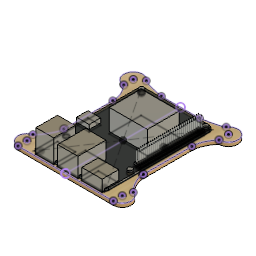
Maaxboard mounted (Autodesk Fusion 360 design; units mm, degrees)
part number: 2026-02-05-11-10-26-845
Autodesk Fusion 360 part; units mm, degrees
sketch "Mount board" plane through (0, 0, 0) normal (0, 0, 1) x (1, 0, 0)
  line L0 (-37.35, 0) -> (37.35, 0)
  line L1 (-31, 90) -> (31, 90)
  line L2 (0, 90) -> (0, 0)
  line L3 (-31, 90) -> (-31, 0)
  line L4 (31, 90) -> (31, 0)
  arc A0 (-39.3579, 13.7058) -> (-37.35, 0) centre (-37.35, 7) ccw
  spline S0 degree 5 poles (-39.3579, 13.7058) (-39.0766, 13.9227) (-38.5354, 14.3685) (-37.7884, 15.0728) (-36.908, 16.081) (-35.9311, 17.4458) (-35.003, 18.9053) (-34.0689, 20.4546) (-33.1263, 22.0975) (-32.2391, 23.848) (-31.5041, 25.7261) (-31.1237, 27.3492) (-30.9957, 28.6435) (-30.986, 29.5419) (-31, 30) knots 0 0 0 0 0 0 0.1 0.2 0.3 0.4 0.5 0.6 0.7 0.8 0.9 1 1 1 1 1 1
  circle A1 centre (-37.35, 7) radius 1.4
  arc A2 (37.35, 0) -> (39.3579, 13.7058) centre (37.35, 7) ccw
  spline S1 degree 5 poles (39.3579, 13.7058) (39.0766, 13.9227) (38.5354, 14.3685) (37.7884, 15.0728) (36.908, 16.081) (35.9311, 17.4458) (35.003, 18.9053) (34.0689, 20.4546) (33.1263, 22.0975) (32.2391, 23.848) (31.5041, 25.7261) (31.1237, 27.3492) (30.9957, 28.6435) (30.986, 29.5419) (31, 30) knots 0 0 0 0 0 0 0.1 0.2 0.3 0.4 0.5 0.6 0.7 0.8 0.9 1 1 1 1 1 1
  line L5 (-40.9476, 12.4803) -> (-37.7683, 14.9314)
  line L6 (-30.9328, 27.8077) -> (-31.0672, 32.1923)
  line L7 (40.9476, 12.4803) -> (37.7683, 14.9314)
  line L8 (30.9328, 27.8077) -> (31.0672, 32.1923)
  circle A3 centre (37.35, 7) radius 1.4
  circle A4 centre (-37.35, 90.3) radius 1.4
  circle A5 centre (-37.35, 90.3) radius 7.4
  spline S2 degree 5 poles (-37.35, 82.9) (-37.1115, 82.6183) (-36.6442, 82.0534) (-35.972, 81.2012) (-35.1342, 80.0554) (-34.1911, 78.606) (-33.3621, 77.1379) (-32.6571, 75.6494) (-32.083, 74.1394) (-31.6366, 72.6084) (-31.3088, 71.0579) (-31.1342, 69.8032) (-31.0494, 68.8545) (-31.0131, 68.2187) (-31, 67.9) knots 0 0 0 0 0 0 0.1 0.2 0.3 0.4 0.5 0.6 0.7 0.8 0.9 1 1 1 1 1 1
  line L9 (-37.35, 82.9) -> (-31, 82.9) construction
  line L10 (-31, 82.9) -> (-31, 67.9) construction
  line L11 (-34.175, 82.9) -> (-31, 82.9) construction
  spline S3 degree 5 poles (-31.2889, 94.5453) (-31.193, 94.4644) (-30.9783, 94.3016) (-30.5874, 94.0544) (-29.9264, 93.7188) (-28.8549, 93.2886) (-27.5267, 92.8473) (-25.9435, 92.3949) (-24.1262, 91.9324) (-22.1003, 91.4609) (-19.891, 90.9814) (-17.9926, 90.5921) (-16.5005, 90.2972) (-15.4759, 90.0993) (-14.9561, 90) knots 0 0 0 0 0 0 0.1 0.2 0.3 0.4 0.5 0.6 0.7 0.8 0.9 1 1 1 1 1 1
  spline S4 degree 5 poles (37.35, 82.9) (37.1115, 82.6183) (36.6442, 82.0534) (35.972, 81.2012) (35.1342, 80.0554) (34.1911, 78.606) (33.3621, 77.1379) (32.6571, 75.6494) (32.083, 74.1394) (31.6366, 72.6084) (31.3088, 71.0579) (31.1342, 69.8032) (31.0494, 68.8545) (31.0131, 68.2187) (31, 67.9) knots 0 0 0 0 0 0 0.1 0.2 0.3 0.4 0.5 0.6 0.7 0.8 0.9 1 1 1 1 1 1
  line L12 (-38.5735, 84.3453) -> (-36.1265, 81.4547)
  line L13 (-31.0729, 69.6717) -> (-30.9271, 66.1283)
  line L14 (38.5735, 84.3453) -> (36.1265, 81.4547)
  line L15 (31.0729, 69.6717) -> (30.9271, 66.1283)
  circle A6 centre (37.35, 90.3) radius 7.4
  circle A7 centre (37.35, 90.3) radius 1.4
  spline S5 degree 5 poles (31.2889, 94.5453) (31.193, 94.4644) (30.9783, 94.3016) (30.5874, 94.0544) (29.9264, 93.7188) (28.8549, 93.2886) (27.5267, 92.8473) (25.9435, 92.3949) (24.1262, 91.9324) (22.1003, 91.4609) (19.891, 90.9814) (17.9926, 90.5921) (16.5005, 90.2972) (15.4759, 90.0993) (14.9561, 90) knots 0 0 0 0 0 0 0.1 0.2 0.3 0.4 0.5 0.6 0.7 0.8 0.9 1 1 1 1 1 1
  line L16 (-32.1151, 95.2425) -> (-30.4626, 93.8481)
  line L17 (-17.1383, 90.4168) -> (-12.7739, 89.5832)
  line L18 (32.1151, 95.2425) -> (30.4626, 93.8481)
  line L19 (17.1383, 90.4168) -> (12.7739, 89.5832)
  point P0 (0, 90)
  point P1 (-34.35, 20)
  point P2 (34.35, 20)
  point P3 (-32.5875, 75.4)
  point P4 (-34.175, 82.9)
  point P5 (-31, 75.4)
  point P6 (-32.5875, 82.9)
  point P7 (-27.9561, 93)
  point P8 (-29.9561, 90)
  point P9 (32.5875, 75.4)
  point P10 (27.9561, 93)
  dimension "d1" = 74.7
  dimension "d2" = 62
  dimension "d3" = 90
  dimension "d4" = 7
  dimension "d5" = 30
  dimension "d6" = 20
  dimension "d7" = 3
  dimension "d8" = 2.8
  dimension "d9" = 2.8
  dimension "d10" = 83.3
  dimension "d11" = 14.8
  dimension "d12" = 15
  dimension "d13" = 15
  dimension "d14" = 3
  dimension "d15" = 2
  constraint horizontal L0
  constraint midpoint L0 L2.end
  constraint coincident L2.end origin
  constraint horizontal L1
  constraint midpoint L1 P0
  constraint coincident P0 L2.start
  constraint coincident L0 L3.end
  constraint perpendicular L0 L3
  constraint coincident L0 L4.end
  constraint perpendicular L0 L4
  constraint tangent L0 A0
  constraint coincident L3 S0.end
  constraint perpendicular L0 L2
  constraint concentric A0 A1
  constraint midpoint A0.start L5
  constraint midpoint S0.end L6
  constraint symmetric L0.start L2 L0.end
  constraint symmetric L2 A0.start A2.end
  constraint symmetric L2 A0 A2
  constraint symmetric L2 P1 P2
  constraint symmetric L2 S0.end S1.end
  constraint symmetric L2 A1 A3
  constraint symmetric L2 L5.start L7.start
  constraint symmetric L2 L5.end L7.end
  constraint symmetric L2 L6.start L8.start
  constraint symmetric L2 L6.end L8.end
  constraint concentric A4 A5
  constraint vertical A0.centre A4.centre
  constraint coincident A5 S2.start
  constraint coincident L3 S2.end
  constraint vertical A4.centre S2.start
  constraint coincident L3 L9.end
  constraint tangent A5 L9
  constraint midpoint L10 P5
  constraint horizontal P3 P5
  constraint coincident P4 L11.start
  constraint perpendicular L3 L11
  constraint midpoint L11 P6
  constraint vertical P3 P6
  constraint coincident A5 S3.start
  constraint coincident L1 S3.end
  constraint coincident L1 P8
  constraint coincident A5 P8
  constraint midpoint S2.start L12
  constraint midpoint S2.end L13
  constraint midpoint S3.start L16
  constraint midpoint S3.end L17
  constraint symmetric L2 A4 A7
  constraint symmetric L2 A5 A6
  constraint symmetric L2 S2.start S4.start
  constraint symmetric L2 P3 P9
  constraint symmetric L2 S2.end S4.end
  constraint symmetric L2 S3.start S5.start
  constraint symmetric L2 P7 P10
  constraint symmetric L2 S3.end S5.end
  constraint symmetric L2 L12.start L14.start
  constraint symmetric L2 L12.end L14.end
  constraint symmetric L2 L13.start L15.start
  constraint symmetric L2 L13.end L15.end
  constraint symmetric L2 L16.start L18.start
  constraint symmetric L2 L16.end L18.end
  constraint symmetric L2 L17.start L19.start
  constraint symmetric L2 L17.end L19.end
  measures "d1" distance of L0.start L0.end
  measures "d2" distance of L1.start L1.end
  measures "d3" distance of L0.start L1
  measures "d4" radius of A0
  measures "d5" distance of L3.end S0.end
  measures "d6" vertical distance of L3.end P1
  measures "d7" horizontal distance of L0.start P1
  measures "d8" diameter of A1
  measures "d9" diameter of A4
  measures "d10" vertical distance of A0.centre A4.centre
  measures "d11" diameter of A5
  measures "d12" distance of S2.end L9.end
  measures "d13" distance of S3.end P8
  measures "d14" vertical distance of P7 P8
  measures "d15" horizontal distance of P7 P8
extrude "Extrude1" add sketch "Mount board" along normal blind 3 contours L0 L3 A0 S0 | L0 L1 L2 L3 S0 A5 | L0 L1 L2 L4 S1 A6 | L0 L4 A2 S1 | L1 A5 S3 | L1 A6 S5 | L3 A5 S2 | L1 L3 A5 | L1 L3 A5 | L1 L4 A6 | L1 L4 A6 | L4 S4 A6 makes body 1
sketch "Sketch2" plane through (0, 0, 3) normal (0, 0, 1) x (-1, 0, 0)
  circle A0 centre (37.35, -90.3) radius 1.4
  circle A1 centre (-37.35, -90.3) radius 1.4
  circle A2 centre (37.35, -7) radius 1.4
  circle A3 centre (-37.35, -7) radius 1.4
  arc A4 (-37.35, -82.9) -> (-31.2889, -94.5453) centre (-37.35, -90.3) ccw
  spline S0 degree 5 poles (-31.2889, -94.5453) (-31.193, -94.4644) (-30.9783, -94.3016) (-30.5874, -94.0544) (-29.9264, -93.7188) (-28.8549, -93.2886) (-27.5267, -92.8473) (-25.9435, -92.3949) (-24.1262, -91.9324) (-22.1003, -91.4609) (-19.891, -90.9814) (-17.9926, -90.5921) (-16.5005, -90.2972) (-15.4759, -90.0993) (-14.9561, -90) knots 0 0 0 0 0 0 0.1 0.2 0.3 0.4 0.5 0.6 0.7 0.8 0.9 1 1 1 1 1 1
  line L0 (-14.9561, -90) -> (14.9561, -90)
  spline S1 degree 5 poles (14.9561, -90) (15.4759, -90.0993) (16.5005, -90.2972) (17.9926, -90.5921) (19.891, -90.9814) (22.1003, -91.4609) (24.1262, -91.9324) (25.9435, -92.3949) (27.5267, -92.8473) (28.8549, -93.2886) (29.9264, -93.7188) (30.5874, -94.0544) (30.9783, -94.3016) (31.193, -94.4644) (31.2889, -94.5453) knots -1 -1 -1 -1 -1 -1 -0.9 -0.8 -0.7 -0.6 -0.5 -0.4 -0.3 -0.2 -0.1 0 0 0 0 0 0
  arc A5 (31.2889, -94.5453) -> (37.35, -82.9) centre (37.35, -90.3) ccw
  spline S2 degree 5 poles (37.35, -82.9) (37.1115, -82.6183) (36.6442, -82.0534) (35.972, -81.2012) (35.1342, -80.0554) (34.1911, -78.606) (33.3621, -77.1379) (32.6571, -75.6494) (32.083, -74.1394) (31.6366, -72.6084) (31.3088, -71.0579) (31.1342, -69.8032) (31.0494, -68.8545) (31.0131, -68.2187) (31, -67.9) knots 0 0 0 0 0 0 0.1 0.2 0.3 0.4 0.5 0.6 0.7 0.8 0.9 1 1 1 1 1 1
  line L1 (31, -67.9) -> (31, -30)
  spline S3 degree 5 poles (31, -30) (30.9948, -29.8295) (30.9922, -29.6602) (30.9922, -29.4921) (30.9948, -29.3252) (31, -29.1596) knots -1 -1 -1 -1 -1 -1 -0.962773 -0.962773 -0.962773 -0.962773 -0.962773 -0.962773
  spline S4 degree 5 poles (31, -29.1596) (31.0088, -28.8804) (31.0505, -28.1652) (31.1963, -27.0481) (31.5588, -25.5863) (32.2391, -23.848) (33.1263, -22.0975) (34.0689, -20.4546) (35.003, -18.9053) (35.9311, -17.4458) (36.908, -16.081) (37.7884, -15.0728) (38.5354, -14.3685) (39.0766, -13.9227) (39.3579, -13.7058) knots -0.962773 -0.962773 -0.962773 -0.962773 -0.962773 -0.962773 -0.9 -0.8 -0.7 -0.6 -0.5 -0.4 -0.3 -0.2 -0.1 0 0 0 0 0 0
  arc A6 (39.3579, -13.7058) -> (37.35, 0) centre (37.35, -7) ccw
  line L2 (37.35, 0) -> (-37.35, 0)
  arc A7 (-37.35, 0) -> (-39.3579, -13.7058) centre (-37.35, -7) ccw
  spline S5 degree 5 poles (-39.3579, -13.7058) (-39.0766, -13.9227) (-38.5354, -14.3685) (-37.7884, -15.0728) (-36.908, -16.081) (-35.9311, -17.4458) (-35.003, -18.9053) (-34.0689, -20.4546) (-33.1263, -22.0975) (-32.2391, -23.848) (-31.5588, -25.5863) (-31.1963, -27.0481) (-31.0505, -28.1652) (-31.0088, -28.8804) (-31, -29.1596) knots 0 0 0 0 0 0 0.1 0.2 0.3 0.4 0.5 0.6 0.7 0.8 0.9 0.962773 0.962773 0.962773 0.962773 0.962773 0.962773
  spline S6 degree 5 poles (-31, -29.1596) (-30.9948, -29.3252) (-30.9922, -29.4921) (-30.9922, -29.6602) (-30.9948, -29.8295) (-31, -30) knots 0.962773 0.962773 0.962773 0.962773 0.962773 0.962773 1 1 1 1 1 1
  line L3 (-31, -30) -> (-31, -67.9)
  spline S7 degree 5 poles (-31, -67.9) (-31.0131, -68.2187) (-31.0494, -68.8545) (-31.1342, -69.8032) (-31.3088, -71.0579) (-31.6366, -72.6084) (-32.083, -74.1394) (-32.6571, -75.6494) (-33.3621, -77.1379) (-34.1911, -78.606) (-35.1342, -80.0554) (-35.972, -81.2012) (-36.6442, -82.0534) (-37.1115, -82.6183) (-37.35, -82.9) knots -1 -1 -1 -1 -1 -1 -0.9 -0.8 -0.7 -0.6 -0.5 -0.4 -0.3 -0.2 -0.1 0 0 0 0 0 0
  line L4 (0, -90) -> (0, 0)
  line L5 (-25.1, -87.5) -> (25.1, -87.5)
  line L6 (28.1, -84.5) -> (28.1, -5.5)
  line L7 (25.1, -2.5) -> (-25.1, -2.5)
  line L8 (-28.1, -5.5) -> (-28.1, -84.5)
  line L9 (-28.1, -87.5) -> (28.1, -2.5) construction
  line L10 (28.1, -87.5) -> (-28.1, -2.5) construction
  arc A8 (25.1, -87.5) -> (28.1, -84.5) centre (25.1, -84.5) ccw
  arc A9 (-28.1, -84.5) -> (-25.1, -87.5) centre (-25.1, -84.5) ccw
  arc A10 (-25.1, -2.5) -> (-28.1, -5.5) centre (-25.1, -5.5) ccw
  arc A11 (28.1, -5.5) -> (25.1, -2.5) centre (25.1, -5.5) ccw
  circle A12 centre (25.1, -84.5) radius 1.875
  circle A13 centre (-25.1, -84.5) radius 1.875
  line L11 (-22.1, -81.5) -> (-22.1, -31.5)
  line L12 (-22.1, -31.5) -> (-27.1, -31.5)
  line L13 (-27.1, -31.5) -> (-27.1, -81.5)
  circle A14 centre (-25.85, -80.7753) radius 0.335
  line L14 (-22.1, -81.5) -> (-24.6, -81.5)
  line L15 (-24.6, -81.5) -> (-27.1, -81.5)
  circle A15 centre (-23.35, -80.7753) radius 0.335
  circle A16 centre (-25.85, -79.2108) radius 0.335
  circle A17 centre (-23.35, -79.2108) radius 0.335
  circle A18 centre (-25.85, -77.6463) radius 0.335
  circle A19 centre (-23.35, -77.6463) radius 0.335
  circle A20 centre (-25.85, -76.0818) radius 0.335
  circle A21 centre (-23.35, -76.0818) radius 0.335
  circle A22 centre (-25.85, -74.5173) radius 0.335
  circle A23 centre (-23.35, -74.5173) radius 0.335
  circle A24 centre (-25.85, -72.9528) radius 0.335
  circle A25 centre (-23.35, -72.9528) radius 0.335
  circle A26 centre (-25.85, -71.3882) radius 0.335
  circle A27 centre (-23.35, -71.3882) radius 0.335
  circle A28 centre (-25.85, -69.8237) radius 0.335
  circle A29 centre (-23.35, -69.8237) radius 0.335
  circle A30 centre (-25.85, -68.2592) radius 0.335
  circle A31 centre (-23.35, -68.2592) radius 0.335
  circle A32 centre (-25.85, -66.6947) radius 0.335
  circle A33 centre (-23.35, -66.6947) radius 0.335
  circle A34 centre (-25.85, -65.1302) radius 0.335
  circle A35 centre (-23.35, -65.1302) radius 0.335
  circle A36 centre (-25.85, -63.5657) radius 0.335
  circle A37 centre (-23.35, -63.5657) radius 0.335
  circle A38 centre (-25.85, -62.0012) radius 0.335
  circle A39 centre (-23.35, -62.0012) radius 0.335
  circle A40 centre (-25.85, -60.4366) radius 0.335
  circle A41 centre (-23.35, -60.4366) radius 0.335
  circle A42 centre (-25.85, -58.8721) radius 0.335
  circle A43 centre (-23.35, -58.8721) radius 0.335
  circle A44 centre (-25.85, -57.3076) radius 0.335
  circle A45 centre (-23.35, -57.3076) radius 0.335
  circle A46 centre (-25.85, -55.7431) radius 0.335
  circle A47 centre (-23.35, -55.7431) radius 0.335
  circle A48 centre (-25.85, -54.1786) radius 0.335
  circle A49 centre (-23.35, -54.1786) radius 0.335
  circle A50 centre (-25.85, -52.6141) radius 0.335
  circle A51 centre (-23.35, -52.6141) radius 0.335
  circle A52 centre (-25.85, -51.0495) radius 0.335
  circle A53 centre (-23.35, -51.0495) radius 0.335
  circle A54 centre (-25.85, -49.485) radius 0.335
  circle A55 centre (-23.35, -49.485) radius 0.335
  circle A56 centre (-25.85, -47.9205) radius 0.335
  circle A57 centre (-23.35, -47.9205) radius 0.335
  circle A58 centre (-25.85, -46.356) radius 0.335
  circle A59 centre (-23.35, -46.356) radius 0.335
  circle A60 centre (-25.85, -44.7915) radius 0.335
  circle A61 centre (-23.35, -44.7915) radius 0.335
  circle A62 centre (-25.85, -43.227) radius 0.335
  circle A63 centre (-23.35, -43.227) radius 0.335
  circle A64 centre (-25.85, -41.6624) radius 0.335
  circle A65 centre (-23.35, -41.6624) radius 0.335
  circle A66 centre (-25.85, -40.0979) radius 0.335
  circle A67 centre (-23.35, -40.0979) radius 0.335
  circle A68 centre (-25.85, -38.5334) radius 0.335
  circle A69 centre (-23.35, -38.5334) radius 0.335
  circle A70 centre (-25.85, -36.9689) radius 0.335
  circle A71 centre (-23.35, -36.9689) radius 0.335
  circle A72 centre (-25.85, -35.4044) radius 0.335
  circle A73 centre (-23.35, -35.4044) radius 0.335
  circle A74 centre (-25.85, -33.8399) radius 0.335
  circle A75 centre (-23.35, -33.8399) radius 0.335
  circle A76 centre (-25.85, -32.2753) radius 0.335
  circle A77 centre (-23.35, -32.2753) radius 0.335
  line L16 (-20.1, -69) -> (9.9, -69)
  line L17 (9.9, -69) -> (9.9, -44)
  line L18 (9.9, -44) -> (-20.1, -44)
  line L19 (-20.1, -44) -> (-20.1, -69)
  line L20 (29.1, -46.5) -> (19.1, -46.5)
  line L21 (19.1, -46.5) -> (19.1, -37.5)
  line L22 (19.1, -37.5) -> (29.1, -37.5)
  line L23 (29.1, -37.5) -> (29.1, -46.5)
  line L24 (-27.1, -14.5) -> (-11.1, -14.5)
  line L25 (-11.1, -14.5) -> (-11.1, -1.5)
  line L26 (-11.1, -1.5) -> (-27.1, -1.5)
  line L27 (-27.1, -1.5) -> (-27.1, -14.5)
  line L28 (-8.1, -1.5) -> (7.9, -1.5)
  line L29 (7.9, -1.5) -> (7.9, -23.5)
  line L30 (7.9, -23.5) -> (-8.1, -23.5)
  line L31 (-8.1, -23.5) -> (-8.1, -1.5)
  line L32 (10.9, -1.5) -> (24.9, -1.5)
  line L33 (24.9, -1.5) -> (24.9, -18.5)
  line L34 (24.9, -18.5) -> (10.9, -18.5)
  line L35 (10.9, -18.5) -> (10.9, -1.5)
  circle A78 centre (-25.1, -25.5) radius 1.875
  circle A79 centre (25.1, -25.5) radius 1.875
  point P0 (0, -45)
  point P1 (0, -45)
  point P2 (-24.6, -81.5)
  point P3 (-23.35, -81.5)
  point P4 (-25.85, -81.5)
  point P5 (-20.1, -56.5)
  point P6 (-22.1, -56.5)
  dimension "d18" = 56.2
  dimension "d19" = 85
  dimension "d20" = 3
  dimension "d22" = 5
  dimension "d23" = 50
  dimension "d25" = 1
  dimension "d26" = 0.67
  dimension "d27" = 0.67
  dimension "d28" = 0.7247
  dimension "d29" = 3
  dimension "d32" = 0
  dimension "d33" = 48.5
  dimension "d34" = 30
  dimension "d35" = 25
  dimension "d36" = 2
  dimension "d37" = 10
  dimension "d38" = 9
  dimension "d39" = 1
  dimension "d40" = 35
  dimension "d41" = 1
  dimension "d42" = 16
  dimension "d43" = 1
  dimension "d44" = 13
  dimension "d45" = 16
  dimension "d46" = 22
  dimension "d48" = 14
  dimension "d49" = 17
  dimension "d50" = 3
  dimension "d51" = 3
  dimension "d52" = 23
  dimension "d53" = 3.75
  constraint midpoint L4 P1
  constraint horizontal L5
  constraint perpendicular L5 L6
  constraint parallel L5 L7
  constraint parallel L6 L8
  constraint coincident L9 P1
  constraint coincident L10 P1
  constraint coincident P1 P0
  constraint coincident L10.start L5
  constraint coincident L10.start L6
  constraint tangent L5 A8
  constraint tangent L6 A8
  constraint coincident L9.start L5
  constraint coincident L9.start L8
  constraint tangent L5 A9
  constraint tangent L8 A9
  constraint equal A8 A9
  constraint coincident L10.end L8
  constraint coincident L10.end L7
  constraint tangent L8 A10
  constraint tangent L7 A10
  constraint equal A8 A10
  constraint coincident L9.end L6
  constraint coincident L9.end L7
  constraint tangent L6 A11
  constraint tangent L7 A11
  constraint equal A8 A11
  constraint concentric A8 A12
  constraint concentric A9 A13
  constraint vertical L11
  constraint horizontal L12
  constraint vertical L13
  constraint coincident P2 L14.end
  constraint midpoint L14 P3
  constraint midpoint L15 P4
  constraint vertical A14.centre P4
  constraint vertical P3 A15.centre
  constraint horizontal A14.centre A15.centre
  constraint perpendicular L11 L14
  constraint perpendicular L13 L15
  constraint equal L14 L15
  constraint horizontal L16
  constraint vertical L17
  constraint horizontal L18
  constraint vertical L19
  constraint midpoint L19 P5
  constraint midpoint L11 P6
  constraint horizontal P5 P6
  constraint horizontal L20
  constraint vertical L21
  constraint horizontal L22
  constraint vertical L23
  constraint horizontal L24
  constraint vertical L25
  constraint horizontal L26
  constraint vertical L27
  constraint horizontal L28
  constraint vertical L29
  constraint horizontal L30
  constraint vertical L31
  constraint horizontal L32
  constraint vertical L33
  constraint horizontal L34
  constraint vertical L35
  constraint collinear L28 L32
  constraint collinear L26 L28
  constraint equal A13 A78
  constraint vertical A9.centre A78.centre
  constraint equal A12 A13
  constraint horizontal A78.centre A79.centre
  constraint vertical A8.centre A79.centre
  constraint equal A78 A79
  measures "d18" distance of L9.end L10.end
  measures "d19" distance of L10.start L9.end
  measures "d20" radius of A8
  measures "d22" distance of L13.end L11.start
  measures "d23" distance of L13.end L12.end
  measures "d25" distance of L8 L13
  measures "d26" diameter of A14
  measures "d27" diameter of A15
  measures "d28" distance of A14.centre L15
  measures "d29" vertical distance of A9.centre P2
  measures "d34" distance of L16.start L16.end
  measures "d35" distance of L16.start L18.end
  measures "d36" distance of L11 L19
  measures "d37" distance of L20.start L20.end
  measures "d38" distance of L20.start L22.end
  measures "d39" distance of L6 L23
  measures "d40" distance of L7 L22
  measures "d41" distance of L7 L32
  measures "d42" distance of L25 L27
  measures "d43" distance of L8 L27
  measures "d44" distance of L24 L26
  measures "d45" distance of L29 L31
  measures "d46" distance of L28.end L29.end
  measures "d48" distance of L33.end L34.end
  measures "d49" distance of L32 L34
  measures "d50" distance of L25 L31
  measures "d51" distance of L29 L35
  measures "d52" distance of L7 A78.centre
  measures "d53" diameter of A12
extrude "Extrude2" add sketch "Sketch2" along normal blind 1.6 separate body contours L4 L5 L7 L8 A9 A10 L16 L18 L19 L24 L25 L27 L30 L31 | L4 L5 L6 L7 A8 A11 L16 L17 L18 L20 L21 L22 L29 L30 L33 L34 L35 makes body 2
extrude "Extrude3" add sketch "Sketch2" along normal blind 18 contours L7 L32 L33 L35 | L7 L33 L34 L35 bodies 2
extrude "Extrude4" add sketch "Sketch2" along normal blind 15 contours L4 L7 L30 L31 | L4 L7 L29 L30 | L4 L7 L28 L29 | L4 L7 L28 L31 bodies 2
extrude "Extrude5" add sketch "Sketch2" along normal blind 9 contours L7 A10 L25 L26 L27 | L7 A10 L24 L25 L27 bodies 2
extrude "Extrude6" add sketch "Sketch2" along normal blind 5 contours L6 L20 L21 L22 | L6 L20 L22 L23 bodies 2
extrude "Extrude7" add sketch "Sketch2" along normal blind 18 contours L4 L16 L18 L19 | L4 L16 L17 L18 bodies 2
extrude "Extrude8" add sketch "Sketch2" along normal blind 12 separate body contours A14 | A15 | A16 | A17 | A18 | A19 | A20 | A21 | A22 | A23 | A24 | A25 | A26 | A27 | A28 | A29 | A30 | A31 | A32 | A33 | A34 | A35 | A36 | A37 | A38 | A39 | A40 | A41 | A42 | A43 | A44 | A45 | A46 | A47 | A48 | A49 | A50 | A51 | A52 | A53 | A54 | A55 | A56 | A57 | A58 | A59 | A60 | A61 | A62 | A63 | A64 | A65 | A66 | A67 | A68 | A69 | A70 | A71 | A72 | A73 | A74 | A75 | A76 | A77 makes body 3 at (25.5154, 65.1135, 7) makes body 4 at (25.5641, 50.8749, 11) makes body 5 at (25.5154, 68.2425, 7) makes body 6 at (25.5641, 61.8265, 11) makes body 7 at (25.5641, 54.0039, 11) makes body 8 at (23.0154, 79.1941, 7) makes body 9 at (23.0154, 77.6296, 7) makes body 10 at (23.0154, 76.0651, 7) makes body 11 at (23.0154, 74.5006, 7) makes body 12 at (25.5641, 49.3103, 11) makes body 13 at (23.0641, 50.8749, 11) makes body 14 at (25.5641, 32.1007, 11) makes body 15 at (25.5641, 35.2297, 11) makes body 16 at (23.0641, 38.3587, 11) makes body 17 at (25.5641, 39.9232, 11) makes body 18 at (25.5641, 41.4878, 11) makes body 19 at (23.0154, 65.1135, 7) makes body 20 at (23.0154, 66.678, 7) makes body 21 at (25.5641, 36.7942, 11) makes body 22 at (23.0641, 35.2297, 11) makes body 23 at (23.0641, 32.1007, 11) makes body 24 at (23.0154, 71.3716, 7) makes body 25 at (23.0154, 72.9361, 7) makes body 26 at (23.0641, 57.1329, 11) makes body 27 at (23.0641, 58.6974, 11) makes body 28 at (23.0641, 60.262, 11) makes body 29 at (23.0641, 61.8265, 11) makes body 30 at (25.5641, 57.1329, 11) makes body 31 at (25.5641, 58.6974, 11) makes body 32 at (25.5154, 79.1941, 7) makes body 33 at (25.5641, 52.4394, 11) makes body 34 at (25.5154, 66.678, 7) makes body 35 at (25.5641, 55.5684, 11) makes body 36 at (25.5154, 71.3716, 7) makes body 37 at (25.5154, 72.9361, 7) makes body 38 at (25.5154, 77.6296, 7) makes body 39 at (23.0641, 43.0523, 11) makes body 40 at (25.5641, 43.0523, 11) makes body 41 at (25.5641, 44.6168, 11) makes body 42 at (25.5641, 46.1813, 11) makes body 43 at (25.5641, 47.7458, 11) makes body 44 at (23.0641, 55.5684, 11) makes body 45 at (23.0641, 52.4394, 11) makes body 46 at (23.0641, 33.6652, 11) makes body 47 at (23.0641, 36.7942, 11) makes body 48 at (25.5641, 38.3587, 11) makes body 49 at (23.0641, 41.4878, 11) makes body 50 at (23.0154, 80.7586, 7) makes body 51 at (25.5154, 80.7586, 7) makes body 52 at (23.0641, 39.9232, 11) makes body 53 at (23.0154, 68.2425, 7) makes body 54 at (25.5641, 33.6652, 11) makes body 55 at (23.0154, 69.807, 7) makes body 56 at (23.0641, 54.0039, 11) makes body 57 at (23.0641, 49.3103, 11) makes body 58 at (23.0641, 47.7458, 11) makes body 59 at (23.0641, 46.1813, 11) makes body 60 at (23.0641, 44.6168, 11) makes body 61 at (23.0641, 63.391, 11) makes body 62 at (25.5641, 60.262, 11) makes body 63 at (25.5154, 76.0651, 7) makes body 64 at (25.5641, 63.391, 11) makes body 65 at (25.5154, 69.807, 7) makes body 66 at (25.5154, 74.5006, 7)
extrude "Extrude9" add sketch "Sketch2" along normal blind 3 contours L11 L12 L13 L14 L15 bodies 2 3 4 5 6 7 8 9 10 11 12 13 14 15 16 17 18 19 20 21 22 23 24 25 26 27 28 29 30 31 32 33 34 35 36 37 38 39 40 41 42 43 44 45 46 47 48 49 50 51 52 53 54 55 56 57 58 59 60 61 62 63 64 65 66
extrude "Extrude10" cut sketch "Sketch2" against normal blind 16 contours A12 | A13 | A78 | A79 bodies 1
extrude "Extrude11" add sketch "Sketch2" along normal blind 3 and the other way blind 5 contours A12 | A13 | A78 | A79 bodies 2
equation "d1 = 77.5 mm - 2.8 mm"
equation "d10 = 86 mm - 2.7 mm"
named bodies: "Mount", "Maaxboard"
